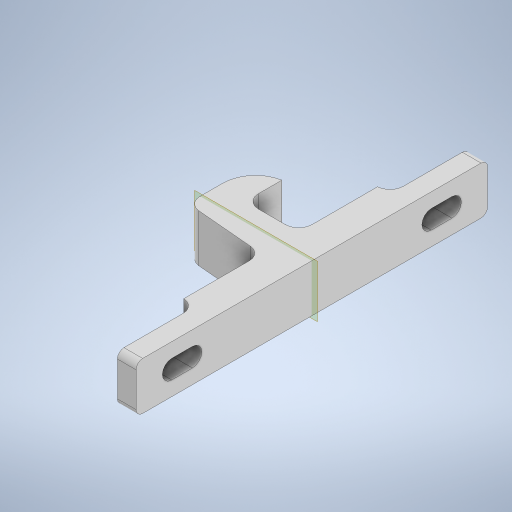
# Autodesk Inventor part: Cierre cocina
Saved by Autodesk Inventor 2024 (Build 280153000, 153)
## iProperties
Created: 2023-08-26
Part Number: Cierre cocina
Material: Genérico
Document SubType Name: Modeling
Designer: sergi
Density: 1 g/cm^3
Appearance: Valor por defecto
Author: sergi
Autodesk Inventor part; units mm, degrees
ref_plane "YZ Plane" through (0, 0, 0) normal (1, 0, 0) x (0, 1, 0)
ref_plane "XZ Plane" through (0, 0, 0) normal (0, 1, 0) x (-1, 0, 0)
ref_plane "XY Plane" through (0, 0, 0) normal (0, 0, 1) x (1, 0, 0)
sketch "Boceto1" plane through (0, 0, 0) normal (0, 1, 0) x (-1, 0, 0)
  line L0 (-2.375, -26.75) -> (2.375, -26.75)
  line L1 (2.375, -26.75) -> (2.375, 26.75)
  line L2 (2.375, 26.75) -> (-2.375, 26.75)
  line L3 (-2.375, 26.75) -> (-2.375, -26.75)
  line L4 (-2.375, -26.75) -> (2.375, 26.75) construction
  line L5 (2.375, -26.75) -> (-2.375, 26.75) construction
  line L6 (2.375, 26.75) -> (0.475, 26.75)
  line L7 (0.475, 26.75) -> (0.475, 14.75)
  line L8 (0.475, 14.75) -> (2.375, 14.75)
  line L9 (2.375, 14.75) -> (2.375, 26.75)
  line L10 (2.375, -26.75) -> (0.475, -26.75)
  line L11 (0.475, -26.75) -> (0.475, -14.75)
  line L12 (0.475, -14.75) -> (2.375, -14.75)
  line L13 (2.375, -14.75) -> (2.375, -26.75)
  line L14 (2.375, -26.75) -> (2.375, -2.75)
  line L15 (2.375, -2.75) -> (10.525, -2.75)
  line L16 (10.525, -2.75) -> (10.525, -8.35)
  line L17 (10.525, -8.35) -> (14.625, -8.35)
  line L18 (14.625, -8.35) -> (14.625, 1.85)
  line L19 (14.625, 1.85) -> (2.375, 1.85)
  line L20 (14.625, 1.85) -> (2.375, 2.9217)
  point P0 (0, 0)
  point P1 (2.375, 14.75)
  point P2 (0.475, -26.75)
  point P3 (2.375, -14.75)
  dimension "d0" = 4.75
  dimension "d1" = 53.5
  dimension "d2" = 1.9
  dimension "d3" = 12
  dimension "d4" = 12
  dimension "d5" = 24
  dimension "d6" = 8.15
  dimension "d7" = 5.6
  dimension "d8" = 4.1
  dimension "d9" = 10.2
  dimension "d10" = 5
  constraints: 42 end point, 7 perpendicular, 6 parallel, 4 point on line, 3 horizontal, 2 midpoint, 1 vertical
  measures "d0" distance of L2.end L1.end
  measures "d1" distance of L0.end L1.end
  measures "d2" distance of L8.end L7.end
  measures "d3" distance of L7.end L6.end
  measures "d4" distance of L10.end L11.end
  measures "d5" distance of L0.end L14.end
  measures "d6" distance of L14.end L15.end
  measures "d7" distance of L15.end L16.end
  measures "d8" distance of L16.end L17.end
  measures "d9" distance of L17.end L18.end
  measures "d10" angle of L19 L20
extrude "Extrusión1" add sketch "Boceto1" along normal blind 7.25 contours L3 L2 L7 L8 L1 L12 L11 L0 | L1 L19 L18 L17 L16 L15 | L1 L20 L19
fillet "Empalme1" radius 2 5 edges at (-0.475, 3.625, -14.75) (-2.375, 3.625, -2.75) (-10.525, 3.625, -2.75) (-2.375, 3.625, 2.9217) (-0.475, 3.625, 14.75)
fillet "Empalme2" radius 2 1 edges at (-14.625, 3.625, 1.85)
fillet "Empalme3" radius 5 1 edges at (-14.625, 3.625, -8.35)
fillet "Empalme4" radius 1 4 edges at (0.95, 7.25, 26.75) (0.95, 0, 26.75) (0.95, 7.25, -26.75) (0.95, 0, -26.75)
sketch "Boceto2" plane through (-0.475, 0, 16.7475) normal (-1, 0, 0) x (0, 0, 1)
  arc A0 (9.0025, 0) -> (10.0025, 1) centre (9.0025, 1) ccw projected
  line L0 (10.0025, 1) -> (10.0025, 6.25) projected
  arc A1 (10.0025, 6.25) -> (9.0025, 7.25) centre (9.0025, 6.25) ccw projected
  line L1 (0, 7.25) -> (9.0025, 7.25) projected
  line L2 (0, 0) -> (0, 7.25) projected
  line L3 (0, 0) -> (9.0025, 0) projected
  arc A2 (-43.4975, 1) -> (-42.4975, 0) centre (-42.4975, 1) ccw projected
  line L4 (-42.4975, 0) -> (-33.495, 0) projected
  line L5 (-33.495, 7.25) -> (-33.495, 0) projected
  line L6 (-42.4975, 7.25) -> (-33.495, 7.25) projected
  arc A3 (-42.4975, 7.25) -> (-43.4975, 6.25) centre (-42.4975, 6.25) ccw projected
  line L7 (-43.4975, 1) -> (-43.4975, 6.25) projected
  line L8 (4.715, 2.2) -> (2.9125, 2.2)
  line L9 (2.2, 5.05) -> (4.5775, 5.05)
  line L10 (10.0025, 3.4658) -> (6.0025, 3.4658)
  line L11 (6.0025, 3.4658) -> (6.0025, 4.2)
  line L12 (6.0025, 3.4658) -> (6.0025, 5.05)
  line L13 (4.5775, 2.2) -> (1.4275, 2.2)
  line L14 (0.0025, 3.625) -> (0.0025, 3.625)
  line L15 (1.4275, 5.05) -> (6.0025, 5.05)
  line L16 (6.0025, 3.625) -> (6.0025, 3.625)
  arc A4 (4.5775, 2.2) -> (6.0025, 3.625) centre (4.5775, 3.625) ccw
  arc A5 (6.0025, 3.625) -> (4.5775, 5.05) centre (4.5775, 3.625) ccw
  arc A6 (1.4275, 5.05) -> (0.0025, 3.625) centre (1.4275, 3.625) ccw
  arc A7 (0.0025, 3.625) -> (1.4275, 2.2) centre (1.4275, 3.625) ccw
  point P0 (-16.7475, 0)
  point P1 (6.0025, 2.2)
  point P2 (0.0025, 5.05)
  point P3 (3.715, 5.05)
  point P4 (0.0025, 3.625)
  point P5 (2.9125, 2.2)
  point P6 (4.5775, 2.2)
  point P7 (2.2, 5.05)
  dimension "d17" = 2.2
  dimension "d18" = 4
  dimension "d19" = 6
  dimension "d21" = 2.85
  dimension "d22" = 1.425
  constraints: 18 end point, 10 point on line, 8 point on circle, 8 tangent, 4 centre point, 3 equal radius, 2 horizontal, 2 parallel, 2 perpendicular, 1 midpoint
  measures "d17" distance between parallel lines of L1 L9
  measures "d18" distance of L10.start L10.end
  measures "d19" distance of L12.end point (0.003, 5.05)
  measures "d21" distance from line of point (3.715, 5.05) L8
  measures "d22" radius of A4
extrude "Extrusión2" cut sketch "Boceto2" against normal blind 7.25 contours L8 L13 A7 A6 L15 L9 A5 A4
ref_plane "Plano de trabajo1" through (2.375, 1, 0) normal (0, 0, -1) x (-1, 0, 0)
mirror "Simetría1" about plane through (2.375, 1, 0) normal (0, 0, -1) of "Extrusión2"
